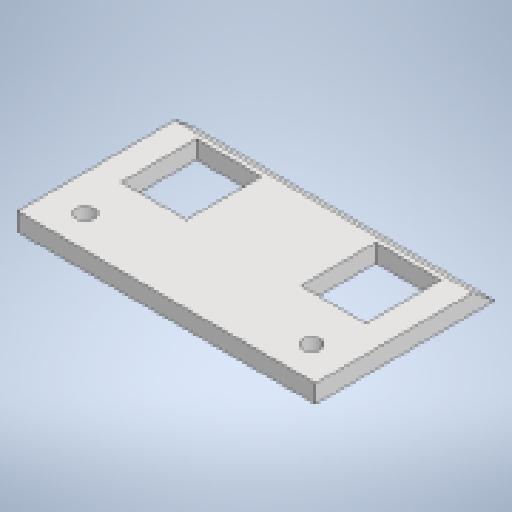
# Autodesk Inventor part: nozz
Saved by Autodesk Inventor 2023 (Build 270158000, 158)
## iProperties
Created: 2023-01-27
Part Number: nozz
Material: Generic
Document SubType Name: Modeling
Designer: Kamil
Density: 1 g/cm^3
Appearance: Default
Author: Kamil
Autodesk Inventor part; units mm, degrees
ref_plane "YZ Plane" through (0, 0, 0) normal (1, 0, 0) x (0, 1, 0)
ref_plane "XZ Plane" through (0, 0, 0) normal (0, 1, 0) x (-1, 0, 0)
ref_plane "XY Plane" through (0, 0, 0) normal (0, 0, 1) x (1, 0, 0)
sketch "Sketch1" plane through (0, 0, 0) normal (1, 0, 0) x (0, 1, 0)
  line L0 (1.944, 4.8709) -> (-1.056, 4.8709)
  line L1 (-1.056, 4.8709) -> (-1.056, -25.1291)
  line L2 (-1.056, -25.1291) -> (1.944, -25.1291)
  line L3 (1.944, -25.1291) -> (1.944, 4.8709)
  line L4 (-1.056, -25.1291) -> (9.6963, -12.315)
  point P0 (0, 0)
  point P1 (1.944, -21.5539)
  dimension "d0" = 3
  dimension "d1" = 30
  dimension "d2" = 40
  constraints: 10 end point, 2 parallel, 1 horizontal, 1 perpendicular
  measures "d0" distance of L2.end L1.end
  measures "d1" distance of L1.end L0.end
  measures "d2" angle of L1 L4
extrude "Extrusion1" add sketch "Sketch1" against normal blind 50 contours L3 L4 L1 L0
sketch "Szkic2" plane through (0, -1.056, -25.1291) normal (0, -1, 0) x (1, 0, 0)
  line L0 (0, 30) -> (0, 0)
  line L1 (0, 30) -> (-50, 30)
  line L2 (-50, 0) -> (-50, 30)
  line L3 (0, 0) -> (-50, 0)
  line L4 (-35.094, 16.557) -> (-35.094, 5.254)
  line L5 (-45, 5) -> (-35.348, 5)
  line L6 (-45, 5) -> (-45, 16.43)
  line L7 (-44.873, 16.557) -> (-35.094, 16.557)
  circle A0 centre (-39.92, 11.35) radius 1
  line L8 (-25, 0) -> (-25, 30)
  line L9 (-35.094, 5.254) -> (-35.348, 5)
  line L10 (-45.5, 16.43) -> (-45.5, 4.5)
  line L11 (-45.5, 4.5) -> (-35.1409, 4.5)
  line L12 (-34.594, 5.0469) -> (-34.594, 17.057)
  line L13 (-34.594, 17.057) -> (-44.873, 17.057)
  line L14 (-35.1409, 4.5) -> (-35.094, 4.5469)
  line L15 (-34.6409, 5) -> (-34.594, 5.0469)
  line L16 (-45.5, 4.5) -> (-34.594, 4.5)
  line L17 (-34.594, 4.5) -> (-34.594, 17.057)
  line L18 (-34.594, 17.057) -> (-45.5, 17.057)
  line L19 (-45.5, 17.057) -> (-45.5, 4.5)
  circle A1 centre (-10.08, 11.35) radius 1
  line L20 (-4.5, 16.43) -> (-4.5, 4.5)
  line L21 (-4.5, 4.5) -> (-14.8591, 4.5)
  line L22 (-15.406, 5.0469) -> (-15.406, 17.057)
  line L23 (-15.406, 17.057) -> (-5.127, 17.057)
  line L24 (-4.5, 4.5) -> (-15.406, 4.5)
  line L25 (-15.406, 4.5) -> (-15.406, 17.057)
  line L26 (-15.406, 17.057) -> (-4.5, 17.057)
  line L27 (-4.5, 17.057) -> (-4.5, 4.5)
  line L28 (0, 4.1492) -> (-50, 4.1492)
  line L29 (-50, 4.1492) -> (-50, 27.66)
  line L30 (-36.5, 27.66) -> (-50, 27.66)
  line L31 (-36.5, 27.66) -> (-36.5, 4.66)
  line L32 (-26.5, 4.66) -> (-36.5, 4.66)
  line L33 (-26.5, 4.66) -> (-26.5, 35.31)
  arc A2 (-26.5, 35.31) -> (-23.5, 35.31) centre (-25, 35.31) ccw
  line L34 (-23.5, 35.31) -> (-23.5, 4.66)
  line L35 (-13.5, 4.66) -> (-23.5, 4.66)
  line L36 (-13.5, 4.66) -> (-13.5, 27.66)
  line L37 (0, 27.66) -> (-13.5, 27.66)
  line L38 (0, 4.1492) -> (0, 27.66)
  line L39 (-50, 4.1492) -> (-44, 4.1492)
  line L40 (-44, 27.66) -> (-50, 27.66)
  line L41 (-50, 27.66) -> (-50, 4.1492)
  line L42 (-50, 27.66) -> (-36.5, 27.66)
  line L43 (-36.5, 27.66) -> (-36.5, 24.66)
  line L44 (-50, 24.66) -> (-50, 27.66)
  circle A3 centre (-10.08, 11.35) radius 1
  circle A4 centre (-39.92, 11.35) radius 1
  line L45 (-6, 27.66) -> (-6, 22.91)
  line L46 (-44, 27.66) -> (-44, 22.91)
  circle A5 centre (-6, 22.91) radius 1.5
  circle A6 centre (-44, 22.91) radius 1.5
  circle A7 centre (-6, 22.91) radius 1.75
  circle A8 centre (-44, 22.91) radius 1.75
  point P0 (0, 25.1291)
extrude "Wyciągnięcie proste2" cut sketch "Szkic2" against normal through all contours L35 L36 L23 L26 L27 L20 L21 L24 L25 | L25 L22 L23 L36 L35 | L32 L31 L5 L9 L4 L7 L13 L12 L17 | L17 L16 L11 L10 L19 L18 L13 L31 L32 | L31 L7 L4 L9 L5 | A0 | A1
sketch "Szkic3" plane through (0, -1.056, -25.1291) normal (0, -1, 0) x (1, 0, 0)
  line L0 (-4.5, 17.057) -> (-4.5, 4.5) projected
  line L1 (-4.5, 4.5) -> (-15.406, 4.5) projected
  line L2 (-15.406, 4.5) -> (-15.406, 17.057) projected
  line L3 (-15.406, 17.057) -> (-4.5, 17.057) projected
  line L4 (-34.594, 17.057) -> (-34.594, 4.5) projected
  line L5 (-34.594, 4.5) -> (-45.5, 4.5) projected
  line L6 (-45.5, 4.5) -> (-45.5, 17.057) projected
  line L7 (-45.5, 17.057) -> (-34.594, 17.057) projected
  line L8 (0, 30) -> (0, 0) projected
  line L9 (0, 30) -> (-50, 30) projected
  line L10 (-50, 0) -> (-50, 30) projected
  line L11 (0, 0) -> (-50, 0) projected
  circle A0 centre (-44, 24.66) radius 1.75 projected
  circle A1 centre (-10.08, 11.35) radius 1 projected
  circle A2 centre (-39.92, 11.35) radius 1 projected
  line L12 (0, 4.1492) -> (-50, 4.1492) projected
  line L13 (-50, 4.1492) -> (-50, 27.66) projected
  line L14 (-36.5, 27.66) -> (-50, 27.66) projected
  line L15 (-36.5, 27.66) -> (-36.5, 4.66) projected
  line L16 (-26.5, 4.66) -> (-36.5, 4.66) projected
  line L17 (-26.5, 4.66) -> (-26.5, 35.31) projected
  arc A3 (-26.5, 35.31) -> (-23.5, 35.31) centre (-25, 35.31) ccw projected
  line L18 (-23.5, 35.31) -> (-23.5, 4.66) projected
  line L19 (-13.5, 4.66) -> (-23.5, 4.66) projected
  line L20 (-13.5, 4.66) -> (-13.5, 27.66) projected
  line L21 (0, 27.66) -> (-13.5, 27.66) projected
  line L22 (0, 4.1492) -> (0, 27.66) projected
  line L23 (-44, 27.66) -> (-44, 22.91)
  line L24 (-6, 27.66) -> (-6, 22.91)
  circle A4 centre (-44, 22.91) radius 1.5
  circle A5 centre (-6, 22.91) radius 1.5
  circle A6 centre (-6, 22.91) radius 1.75 projected
  circle A7 centre (-44, 22.91) radius 1.75 projected
  point P0 (0, 25.1291)
  dimension "d13" = 3
  dimension "d14" = 3
  constraints: 4 end point, 2 centre point, 2 coincident, 2 point on line, 1 perpendicular
  measures "d13" diameter of A4
  measures "d14" diameter of A5
extrude "Wyciągnięcie proste3" cut sketch "Szkic3" against normal through all contours A4 A0 | A0 L23 A4 | A4 L23 A0 | A5
body "Solid1"
